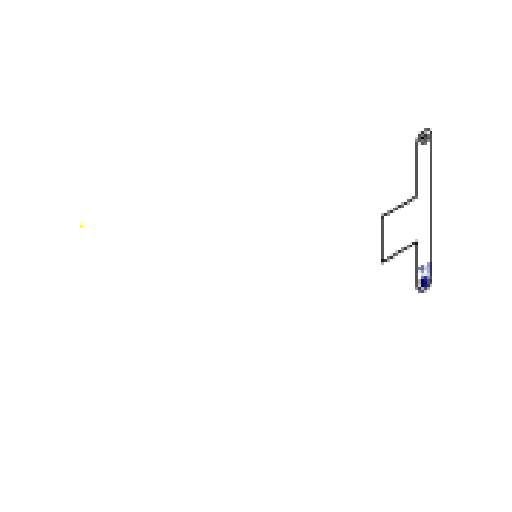
# Autodesk Inventor part: VertialIntakeSlides
Saved by Autodesk Inventor 2023 (Build 270158000, 158)
## iProperties
Created: 2022-11-08
Part Number: VertialIntakeSlides
Material: Generic
Document SubType Name: Modeling
Designer: deli
Density: 1 g/cm^3
Appearance: Default
Author: deli
Autodesk Inventor part; units mm, degrees
ref_plane "YZ Plane" through (0, 0, 0) normal (1, 0, 0) x (0, 1, 0)
ref_plane "XZ Plane" through (0, 0, 0) normal (0, 1, 0) x (-1, 0, 0)
ref_plane "XY Plane" through (0, 0, 0) normal (0, 0, 1) x (1, 0, 0)
sketch "Sketch1" plane through (0, 0, 0) normal (1, 0, 0) x (0, 1, 0)
  line L0 (-11.9114, -190.7198) -> (-51.9114, -190.7198)
  line L1 (-51.9114, -190.7198) -> (-51.9114, -181.7198)
  line L2 (-51.9114, -181.7198) -> (-65.4114, -181.7198)
  line L3 (-65.4114, -181.7198) -> (-65.4114, -190.7198)
  line L4 (-65.4114, -190.7198) -> (-125.4114, -190.7198)
  arc A0 (-11.9114, -198.7198) -> (-11.9114, -190.7198) centre (-11.9114, -194.7198) ccw
  arc A1 (-125.4114, -190.7198) -> (-125.4114, -198.7198) centre (-125.4114, -194.7198) ccw
  line L5 (-11.9114, -198.7198) -> (-125.4114, -198.7198)
  circle A2 centre (-125.4114, -194.7198) radius 2
  circle A3 centre (-11.9114, -194.7198) radius 2
  circle A4 centre (-54.6614, -184.2198) radius 1.1
  circle A5 centre (-54.6614, -196.2198) radius 1.1
  circle A6 centre (-62.6614, -184.2198) radius 1.1
  circle A7 centre (-62.6614, -196.2198) radius 1.1
  line L6 (-54.6614, -184.2198) -> (-62.6614, -184.2198) construction
  line L7 (-62.6614, -184.2198) -> (-62.6614, -196.2198) construction
  line L8 (-62.6614, -196.2198) -> (-54.6614, -196.2198) construction
  line L9 (-54.6614, -196.2198) -> (-54.6614, -184.2198) construction
  circle A8 centre (-109.4114, -194.7198) radius 2
  point P0 (0, 0)
  dimension "d0" = 8
  dimension "d1" = 4
  dimension "d2" = 13.5
  dimension "d3" = 17
  dimension "d4" = 2.2
  dimension "d5" = 12
  dimension "d6" = 8
  dimension "d7" = 2.75
  dimension "d8" = 2.5
  dimension "d9" = 4
  dimension "d10" = 16
  dimension "d11" = 60
  dimension "d12" = 40
  constraints: 20 end point, 9 centre point, 6 equal radius, 5 perpendicular, 4 point on circle, 3 horizontal, 3 tangent, 2 coincident, 2 point on line, 1 parallel
  measures "d0" diameter of A1
  measures "d1" diameter of A2
  measures "d2" distance between parallel lines of L3 L1
  measures "d3" distance between parallel lines of L5 L2
  measures "d4" diameter of A4
  measures "d5" distance of L8.end L6.start
  measures "d6" distance of L6.start L6.end
  measures "d7" distance between parallel lines of L3 L7
  measures "d8" distance between parallel lines of L2 L6
  measures "d9" distance from line of L5 A8.centre
  measures "d10" distance of A2.centre A8.centre
  measures "d11" distance of L3.end L4.end
  measures "d12" distance of L0.start L0.end
extrude "Extrusion1" add sketch "Sketch1" along normal blind 3.175
equation "\"d7\" = -0.5 * d6 + 0.5 * d2"
equation "\"d8\" = -0.5 * d5 + 0.5 * d3"
equation "\"d9\" = 0.5 * d0"
body "Solid1"
